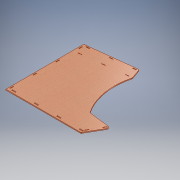
# Autodesk Inventor part: ladoA
Saved by Autodesk Inventor 2017 (Build 210142000, 142)
## iProperties
Created: 2017-10-02
Part Number: ladoA
Material: Wood (Oak)
Document SubType Name: Modeling
Designer: Felipe
Density: 0.76 g/cm^3
Appearance: White Oak - Natural Medium Gloss
Author: Felipe
Autodesk Inventor part; units mm, degrees
ref_plane "YZ Plane" through (0, 0, 0) normal (1, 0, 0) x (0, 1, 0)
ref_plane "XZ Plane" through (0, 0, 0) normal (0, 1, 0) x (-1, 0, 0)
ref_plane "XY Plane" through (0, 0, 0) normal (0, 0, 1) x (1, 0, 0)
sketch "Sketch1" plane through (0, 0, 0) normal (0, 0, 1) x (1, 0, 0)
  line L0 (0, 0) -> (794.2265, 0)
  line L1 (0, 0) -> (0, 821.1016)
  line L2 (8.8381, 831.0339) -> (522.0969, 891.0755)
  line L3 (802.8868, 5) -> (900.3166, 173.7534)
  line L4 (532.6762, 884.5066) -> (567.9402, 785.7674)
  arc A0 (532.6762, 884.5066) -> (522.0969, 891.0755) centre (523.2588, 881.1432) ccw
  arc A1 (8.8381, 831.0339) -> (0, 821.1016) centre (10, 821.1016) ccw
  arc A2 (794.2265, 0) -> (802.8868, 5) centre (794.2265, 10) ccw
  line L5 (265.4675, 861.0547) -> (267.2222, 846.0547) construction
  line L6 (14.3861, 816.4776) -> (535.2127, 877.4045) construction
  line L7 (20, 820.1548) -> (531.512, 879.9921) construction
  line L8 (531.512, 879.9921) -> (532.2091, 874.0327) construction
  line L9 (532.2091, 874.0327) -> (20.6971, 814.1954) construction
  line L10 (20.6971, 814.1954) -> (20, 820.1548) construction
  line L11 (34.8984, 821.8976) -> (35.5955, 815.9383)
  line L12 (69.6614, 825.9643) -> (70.3585, 820.0049)
  line L13 (481.8506, 874.1826) -> (482.5478, 868.2233)
  line L14 (516.6136, 878.2492) -> (517.3107, 872.2899)
  line L15 (34.8984, 821.8976) -> (69.6614, 825.9643)
  line L16 (70.3585, 820.0049) -> (35.5955, 815.9383)
  line L17 (516.6136, 878.2492) -> (481.8506, 874.1826)
  line L18 (482.5478, 868.2233) -> (517.3107, 872.2899)
  line L19 (20.3486, 817.1751) -> (531.8605, 877.0124) construction
  line L20 (275.756, 850.0734) -> (276.1046, 847.0938) construction
  line L21 (569.7285, 780.7603) -> (0, 714.1128) construction
  line L22 (49.9711, 721.4687) -> (50.3197, 718.489)
  line L23 (84.734, 725.5353) -> (85.0826, 722.5557)
  line L24 (501.8894, 774.3347) -> (502.238, 771.355)
  line L25 (536.6524, 778.4013) -> (537.001, 775.4216)
  line L26 (49.9711, 721.4687) -> (84.734, 725.5353)
  line L27 (85.0826, 722.5557) -> (50.3197, 718.489)
  line L28 (536.6524, 778.4013) -> (501.8894, 774.3347)
  line L29 (502.238, 771.355) -> (537.001, 775.4216)
  line L30 (20, 719.4729) -> (566.2749, 783.3768) construction
  line L31 (566.2749, 783.3768) -> (566.9721, 777.4174) construction
  line L32 (566.9721, 777.4174) -> (20.6971, 713.5135) construction
  line L33 (20.6971, 713.5135) -> (20, 719.4729) construction
  line L34 (15, 0) -> (15, 541.5516) construction
  line L35 (12, 800) -> (18, 800)
  line L36 (18, 800) -> (18, 765)
  line L37 (18, 765) -> (12, 765)
  line L38 (12, 765) -> (12, 800)
  line L39 (12, 555) -> (18, 555)
  line L40 (18, 555) -> (18, 520)
  line L41 (18, 520) -> (12, 520)
  line L42 (12, 520) -> (12, 555)
  line L43 (12, 310) -> (18, 310)
  line L44 (18, 310) -> (18, 275)
  line L45 (18, 275) -> (12, 275)
  line L46 (12, 275) -> (12, 310)
  line L47 (12, 65) -> (18, 65)
  line L48 (18, 65) -> (18, 30)
  line L49 (18, 30) -> (12, 30)
  line L50 (12, 30) -> (12, 65)
  line L51 (31.6599, 656.3688) -> (531.6599, 656.3688) construction
  line L52 (531.6599, 656.3688) -> (531.6599, 36.3688) construction
  line L53 (531.6599, 36.3688) -> (31.6599, 36.3688) construction
  line L54 (31.6599, 36.3688) -> (31.6599, 656.3688) construction
  line L55 (885.379, 203.6109) -> (674.5616, 228.909)
  arc A3 (568.4993, 774.1544) -> (660.278, 237.7109) centre (1221.1056, 609.7342) ccw
  line L56 (40, 30) -> (80, 30)
  line L57 (80, 30) -> (80, 20)
  line L58 (80, 20) -> (40, 20)
  line L59 (40, 20) -> (40, 30)
  line L60 (280, 30) -> (320, 30)
  line L61 (320, 30) -> (320, 20)
  line L62 (320, 20) -> (280, 20)
  line L63 (280, 20) -> (280, 30)
  line L64 (520, 30) -> (560, 30)
  line L65 (560, 30) -> (560, 20)
  line L66 (560, 20) -> (520, 20)
  line L67 (520, 20) -> (520, 30)
  line L68 (760, 30) -> (800, 30)
  line L69 (800, 30) -> (800, 20)
  line L70 (800, 20) -> (760, 20)
  line L71 (760, 20) -> (760, 30)
  arc A4 (900.3166, 173.7534) -> (885.379, 203.6109) centre (882.9961, 183.7534) ccw
  arc A5 (660.278, 237.7109) -> (674.5616, 228.909) centre (676.9445, 248.7665) ccw
  arc A6 (568.4993, 774.1544) -> (567.9402, 785.7674) centre (549.1054, 779.0406) ccw
  line L72 (52.2799, 823.9309) -> (52.6284, 820.9513) construction
  line L73 (258.6126, 846.0051) -> (259.0716, 842.0808)
  line L74 (293.3755, 850.0717) -> (293.8346, 846.1474)
  line L75 (258.6126, 846.0051) -> (293.3755, 850.0717)
  line L76 (293.8346, 846.1474) -> (259.0716, 842.0808)
  line L77 (275.994, 848.0384) -> (276.3426, 845.0587) construction
  line L78 (519.2709, 776.368) -> (519.4452, 774.8781)
  line L79 (310.1966, 751.9102) -> (310.5452, 748.9305)
  line L80 (275.4337, 747.8436) -> (275.7822, 744.8639)
  line L81 (310.1966, 751.9102) -> (275.4337, 747.8436)
  line L82 (275.7822, 744.8639) -> (310.5452, 748.9305)
  line L83 (292.8151, 749.8769) -> (292.9894, 748.3871)
  line L84 (796.8079, 40.4711) -> (802.0041, 37.4711)
  line L85 (802.0041, 37.4711) -> (819.5041, 67.782)
  line L86 (819.5041, 67.782) -> (814.3079, 70.782)
  line L87 (814.3079, 70.782) -> (796.8079, 40.4711)
  line L88 (873.5041, 161.3128) -> (868.3079, 164.3128)
  line L89 (868.3079, 164.3128) -> (885.8079, 194.6237)
  line L90 (885.8079, 194.6237) -> (891.0041, 191.6237)
  line L91 (891.0041, 191.6237) -> (873.5041, 161.3128)
  line L92 (840.6385, 70.388) -> (823.318, 80.388) construction
  line L93 (892.9961, 201.0739) -> (776.906, 0) construction
  line L94 (799.406, 38.9711) -> (888.406, 193.1237) construction
  line L95 (843.906, 116.0474) -> (847.4398, 114.0072) construction
  line L96 (797.981, 30.503) -> (792.7848, 33.503) construction
  line L97 (796.8079, 40.4711) -> (792.7848, 33.503) construction
  line L98 (801.8634, 37.2275) -> (797.981, 30.503) construction
  line L99 (819.5041, 67.782) -> (873.5041, 161.3128) construction
  line L100 (868.3079, 164.3128) -> (814.3079, 70.782) construction
  line L101 (885.8079, 194.6237) -> (890.2848, 202.3779) construction
  line L102 (891.0041, 191.6237) -> (895.481, 199.3779) construction
  line L103 (890.2848, 202.3779) -> (895.481, 199.3779) construction
  line L104 (569.0823, 778.0788) -> (665.4701, 230) construction
  line L105 (665.4701, 230) -> (546.1008, 230) construction
  line L106 (569.0823, 778.0788) -> (515.1258, 778.0788) construction
  line L107 (509.3451, 770.6761) -> (604.6809, 230) construction
  point P0 (800, 0)
  point P1 (0, 830)
  point P2 (530, 892)
  point P3 (570, 780)
  point P4 (915.4701, 200)
  point P5 (570, 780)
  point P6 (15, 65)
  point P7 (84.9083, 724.0455)
  point P8 (502.0637, 772.8448)
  point P9 (20.3486, 716.4932)
  point P10 (275.6079, 746.3538)
  dimension "d0" = 830
  dimension "d1" = 62
  dimension "d2" = 50
  dimension "d3" = 800
  dimension "d9" = 530
  dimension "d10" = 570
  dimension "d13" = 10
  dimension "d16" = 15
  dimension "d17" = 6
  dimension "d18" = 515
  dimension "d19" = 35
  dimension "d20" = 15
  dimension "d21" = 15
  dimension "d22" = 35
  dimension "d23" = 415
  dimension "d24" = 35
  dimension "d25" = 35
  dimension "d27" = 6
  dimension "d28" = 550
  dimension "d31" = 15
  dimension "d32" = 35
  dimension "d33" = 6
  dimension "d34" = 30
  dimension "d35" = 210
  dimension "d36" = 210
  dimension "d37" = 210
  dimension "d38" = 30
  dimension "d39" = 30
  dimension "d40" = 420
  dimension "d42" = 20
  dimension "d48" = 3
  dimension "d50" = 5
  dimension "d51" = 100
  dimension "d58" = 500
  dimension "d59" = 620
  dimension "d60" = 200
  dimension "d61" = 230
  dimension "d62" = 250
  dimension "d63" = 10
  dimension "d64" = 40
  dimension "d65" = 200
  dimension "d66" = 200
  dimension "d67" = 200
  dimension "d68" = 40
  dimension "d69" = 20
  dimension "d72" = 20
  dimension "d73" = 35
  dimension "d74" = 20
  dimension "d75" = 20
  dimension "d76" = 10
  dimension "d77" = 35
  dimension "d78" = 192
  dimension "d79" = 193
  dimension "d80" = 673
  dimension "d84" = 22
  dimension "d85" = 190
  dimension "d86" = 190
  dimension "d87" = 6
  dimension "d88" = 35
  dimension "d89" = 20
  dimension "d90" = 120
  dimension "d91" = 45
  dimension "d92" = 108
  dimension "d93" = 195
  constraints: 216 end point, 49 point on line, 38 parallel, 27 perpendicular, 19 point on circle, 18 midpoint, 13 tangent, 12 horizontal, 10 equal length, 8 collinear, 7 centre point, 4 equal radius, 2 vertical, 1 coincident
  measures "d0" distance of L0.start point (0, 830)
  measures "d1" vertical distance of point (0, 830) point (530, 892)
  measures "d2" vertical distance of point (570, 780) point (0, 830)
  measures "d3" distance of L0.start point (800, 0)
  measures "d9" distance from line of point (530, 892) L1
  measures "d10" distance from line of point (570, 780) L1
  measures "d13" radius of A0
  measures "d16" vertical distance of L5.start L5.end
  measures "d17" distance of L9.end L7.start
  measures "d18" distance of L7.start L7.end
  measures "d19" distance of L11.start L12.start
  measures "d20" distance between parallel lines of L10 L11
  measures "d21" distance between parallel lines of L8 L14
  measures "d22" distance between parallel lines of L14 L13
  measures "d23" distance between parallel lines of L12 L13
  measures "d24" distance of L26.start L23.start
  measures "d25" distance between parallel lines of L25 L24
  measures "d27" distance of L33.start L30.start
  measures "d28" distance of L30.start L30.end
  measures "d31" distance between parallel lines of L1 L34
  measures "d32" distance of L47.end L48.end
  measures "d33" distance of L48.end L49.end
  measures "d34" distance between parallel lines of L0 L49
  measures "d35" distance between parallel lines of L47 L45
  measures "d36" distance between parallel lines of L41 L43
  measures "d37" distance between parallel lines of L37 L39
  measures "d38" distance between parallel lines of L33 L22
  measures "d39" distance between parallel lines of L31 L25
  measures "d40" distance between parallel lines of L24 L23
  measures "d42" distance from line of L1 L7.start
  measures "d48" distance between parallel lines of L27 L26
  measures "d50" distance from line of L34 L30.start
  measures "d51" distance between parallel lines of L21 L19
  measures "d58" distance of L51.start L51.end
  measures "d59" distance of L53.end L51.start
  measures "d60" distance from line of L0 point (915.47, 200)
  measures "d61" distance from line of L0 L104.end
  measures "d62" horizontal distance of point (915.47, 200) L104.end
  measures "d63" distance of L58.end L56.start
  measures "d64" distance of L56.start L56.end
  measures "d65" distance between parallel lines of L71 L65
  measures "d66" distance between parallel lines of L67 L61
  measures "d67" distance between parallel lines of L57 L63
  measures "d68" distance between parallel lines of L1 L59
  measures "d69" distance between parallel lines of L0 L58
  measures "d72" radius of A4
  measures "d73" distance of L73.start L74.start
  measures "d74" radius of A6
  measures "d75" radius of A5
  measures "d76" radius of A2
  measures "d77" distance between parallel lines of L79 L80
  measures "d78" distance between parallel lines of L23 L80
  measures "d79" distance between parallel lines of L24 L79
  measures "d80" radius of A3
  measures "d84" distance between parallel lines of L48 L59
  measures "d85" distance between parallel lines of L12 L73
  measures "d86" distance between parallel lines of L13 L74
  measures "d87" distance of L85.end L86.end
  measures "d88" distance of L84.end L85.end
  measures "d89" distance between parallel lines of L3 L93
  measures "d90" angle of L0 L93
  measures "d91" distance from line of L93.end L84
  measures "d92" distance between parallel lines of L88 L86
  measures "d93" distance between parallel lines of L103 L96
extrude "Extrusion6" add sketch "Sketch1" along normal blind 10
body "Solid6"
